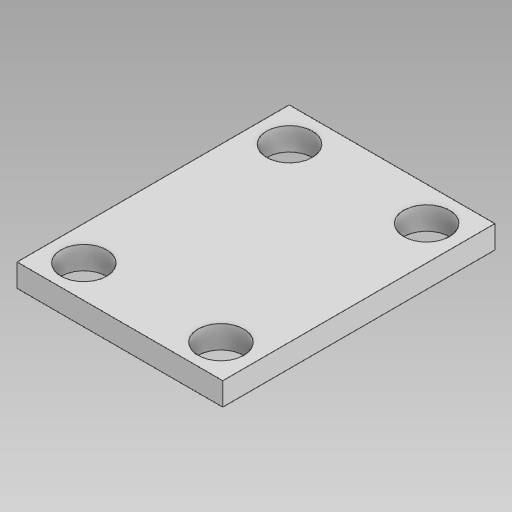
# Autodesk Inventor part: XL_XL_interface
Saved by Autodesk Inventor 2021 (Build 250183000, 183)
## iProperties
Created: 2020-11-15
Part Number: XL_XL_interface
Material: Generic
Document SubType Name: Modeling
Designer: Paco
Density: 1 g/cm^3
Appearance: Default
Mass: 0.756828 g
Surface Area: 10.2462 cm^2
Volume: 0.756828 cm^3
Author: Paco
Autodesk Inventor part; units mm, degrees
ref_plane "YZ Plane" through (0, 0, 0) normal (1, 0, 0) x (0, 1, 0)
ref_plane "XZ Plane" through (0, 0, 0) normal (0, 1, 0) x (-1, 0, 0)
ref_plane "XY Plane" through (0, 0, 0) normal (0, 0, 1) x (1, 0, 0)
sketch "Sketch1" plane through (0, 0, 0) normal (0, 1, 0) x (-1, 0, 0)
  line L0 (-6, 5.8405) -> (-12, 5.8405)
  line L1 (6, -17.975) -> (6, -12)
  line L2 (-12, 5.8405) -> (6, 5.8405)
  line L3 (6, 5.8405) -> (6, -17.975)
  line L4 (6, -17.975) -> (-12, -17.975)
  line L5 (-12, -17.975) -> (-12, 5.8405)
  circle A0 centre (-9, 3) radius 2
  circle A1 centre (-9, 3) radius 2
  circle A2 centre (3, 3) radius 2
  circle A3 centre (3, 3) radius 2
  circle A4 centre (3, -15) radius 2
  circle A5 centre (3, -15) radius 2
  circle A6 centre (-9, -15) radius 2
  point P0 (-3, 3)
  dimension "d2" = 12
  constraints: 12 end point, 7 centre point, 3 coincident, 2 parallel, 1 horizontal, 1 perpendicular
  measures "d2" distance of A6.centre A5.centre
extrude "Extrusion1" add sketch "Sketch1" along normal blind 2
body "Solid1"
